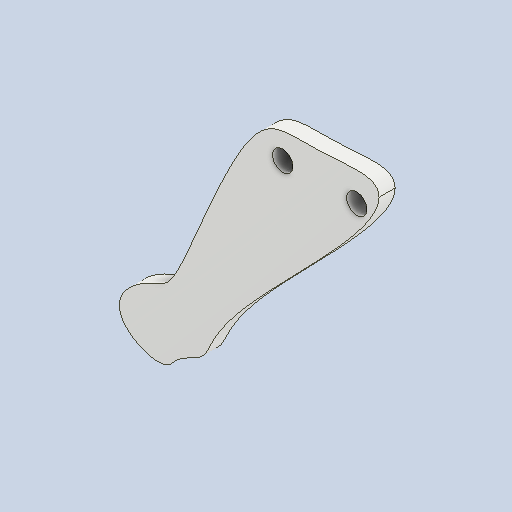
# Autodesk Inventor part: Component30
Saved by Autodesk Inventor 2022 (Build 260153000, 153)
## iProperties
Created: 2022-01-29
Part Number: Component30
Material: Generic
Document SubType Name: Modeling
Designer: Administrator
Density: 1 g/cm^3
Appearance: Default
Title: Component30
Author: Administrator
Autodesk Inventor part; units mm, degrees
ref_plane "YZ Plane" through (0, 0, 0) normal (1, 0, 0) x (0, 1, 0)
ref_plane "XZ Plane" through (0, 0, 0) normal (0, 1, 0) x (-1, 0, 0)
ref_plane "XY Plane" through (0, 0, 0) normal (0, 0, 1) x (1, 0, 0)
sketch "Sketch2" plane through (0, 0, 0) normal (0, 0, 1) x (1, 0, 0)
  circle A0 centre (35.9634, 27.435) radius 3.175
  circle A1 centre (12.8806, 27.4768) radius 3.175
  spline S0 degree 5 poles (42.9087, 32.6199) (42.9087, 31.9081) (42.6577, 30.3121) (41.5232, 27.4166) (38.5767, 22.7043) (32.9176, 15.7206) (25.8984, 8.057) (18.2235, 0.12) (10.6186, -7.6858) (3.7431, -14.995) (-1.8875, -21.5012) (-5.9876, -26.9846) (-8.5758, -31.3344) (-10.0791, -34.5811) (-11.2129, -36.8809) (-12.6292, -38.4862) (-14.9015, -39.7158) (-17.6495, -40.9387) (-19.9276, -42.4221) (-21.3165, -44.1568) (-22.6552, -45.7102) (-25.1043, -46.494) (-28.9667, -46.0656) (-33.4217, -44.2668) (-37.1421, -41.1877) (-38.8028, -37.1756) (-37.3333, -32.8308) (-33.5057, -29.0054) (-28.9893, -26.3383) (-25.4052, -24.9519) (-23.2034, -23.8632) (-21.0247, -20.9963) (-18.4454, -15.8053) (-15.2035, -8.349) (-11.3737, 0.6639) (-7.1563, 10.2254) (-2.8343, 19.2022) (1.3468, 26.5978) (5.2526, 31.7475) (8.9887, 34.6167) (12.8504, 35.7307) (17.1606, 35.8645) (22.131, 35.7893) (27.7338, 36.027) (33.5168, 36.5248) (38.6536, 36.6756) (41.5325, 35.9263) (42.6577, 34.5828) (42.9087, 33.3317) (42.9087, 32.6199) knots 0 0 0 0 0 0 0.022222 0.044444 0.066667 0.088889 0.111111 0.133333 0.155556 0.177778 0.2 0.222222 0.244444 0.266667 0.288889 0.311111 0.333333 0.355556 0.377778 0.4 0.422222 0.444444 0.466667 0.488889 0.511111 0.533333 0.555556 0.577778 0.6 0.622222 0.644444 0.666667 0.688889 0.711111 0.733333 0.755556 0.777778 0.8 0.822222 0.844444 0.866667 0.888889 0.911111 0.933333 0.955556 0.977778 1 1 1 1 1 1 weights 1 1 1 1 1 1 1 1 1 1 1 1 1 1 1 1 1 1 1 1 1 1 1 1 1 1 1 1 1 1 1 1 1 1 1 1 1 1 1 1 1 1 1 1 1 1 1 1 1 1
  point P0 (0, 0)
  point P1 (-99.0292, 92.9189)
  constraints: 2 centre point, 1 other
extrude "Extrusion1" add sketch "Sketch2" along normal blind 5
body "Solid1"
